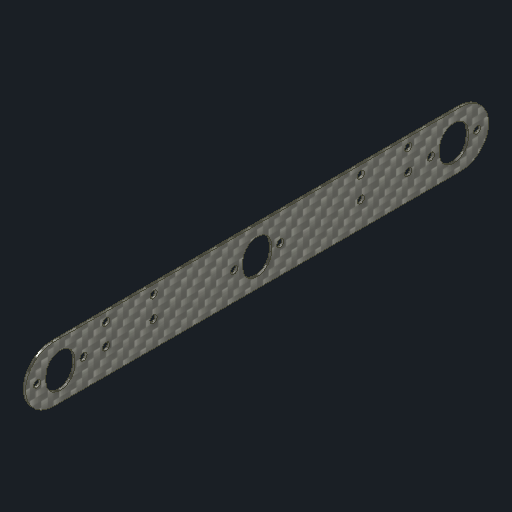
# Autodesk Inventor part: Leg_Loadpipe_Plate_Inner
Saved by Autodesk Inventor 2024.1 (Build 281209000, 209)
## iProperties
Created: 2023-06-16
Part Number: Leg_Loadpipe_Plate_Inner
Material: CFRP
Document SubType Name: Modeling
Designer: dzw04
Density: 1.43 g/cm^3
Appearance: Carbon Fiber 1
Author: dzw04
Autodesk Inventor part; units mm, degrees
ref_plane "YZ Plane" through (0, 0, 0) normal (1, 0, 0) x (0, 1, 0)
ref_plane "XZ Plane" through (0, 0, 0) normal (0, 1, 0) x (-1, 0, 0)
ref_plane "XY Plane" through (0, 0, 0) normal (0, 0, 1) x (1, 0, 0)
sketch "Sketch1" plane through (0, 0, 0) normal (1, 0, 0) x (0, 1, 0)
  line L0 (-1.25, 6.25) -> (1.25, 6.25)
  arc A0 (1.25, -6.25) -> (1.25, 6.25) centre (1.25, 0) ccw
  line L1 (1.25, -6.25) -> (-1.25, -6.25)
  arc A1 (-1.25, 6.25) -> (-1.25, -6.25) centre (-1.25, 0) ccw
  circle A2 centre (0, -10) radius 1.6
  circle A3 centre (0, 10) radius 1.6
  circle A4 centre (8.25, 44.75) radius 1.6
  circle A5 centre (8.25, 65.25) radius 1.6
  line L2 (-1.25, 91.25) -> (1.25, 91.25)
  arc A6 (1.25, 78.75) -> (1.25, 91.25) centre (1.25, 85) ccw
  line L3 (1.25, 78.75) -> (-1.25, 78.75)
  arc A7 (-1.25, 91.25) -> (-1.25, 78.75) centre (-1.25, 85) ccw
  circle A8 centre (0, 75) radius 1.6
  circle A9 centre (0, 95) radius 1.6
  line L4 (-1.25, -91.25) -> (1.25, -91.25)
  arc A10 (1.25, -91.25) -> (1.25, -78.75) centre (1.25, -85) ccw
  line L5 (1.25, -78.75) -> (-1.25, -78.75)
  arc A11 (-1.25, -78.75) -> (-1.25, -91.25) centre (-1.25, -85) ccw
  circle A12 centre (0, -75) radius 1.6
  circle A13 centre (0, -95) radius 1.6
  circle A14 centre (-0.972, 44.75) radius 1.6
  circle A15 centre (-0.972, 65.25) radius 1.6
  circle A16 centre (8.25, -44.75) radius 1.6
  circle A17 centre (8.25, -65.25) radius 1.6
  circle A18 centre (-0.972, -44.75) radius 1.6
  circle A19 centre (-0.972, -65.25) radius 1.6
  arc A20 (12, 88) -> (-12, 88) centre (0, 88) ccw
  line L6 (12, 88) -> (12, -88)
  arc A21 (-12, -88) -> (12, -88) centre (0, -88) ccw
  line L7 (-12, -88) -> (-12, 88)
  point P0 (0, 0)
  point P1 (0, 0)
  point P2 (-12, -88)
  point P3 (12, 88)
  point P4 (-12, 88)
  point P5 (1.25, -78.75)
  point P6 (1.25, 78.75)
  point P7 (-1.25, 78.75)
  point P8 (1.25, -6.25)
  point P9 (-1.25, -6.25)
  dimension "d2" = 3.2
  dimension "d3" = 3.2
  dimension "d4" = 3.2
  dimension "d5" = 3.2
  dimension "d6" = 9.222
  dimension "d7" = 9.222
  dimension "d8" = 9.222
  dimension "d11" = 3.2
  dimension "d12" = 3.2
  dimension "d13" = 3.2
  dimension "d14" = 3.2
  dimension "d15" = 3.2
  dimension "d16" = 3.2
  dimension "d17" = 3.2
  dimension "d18" = 3.2
  dimension "d19" = 3.2
  dimension "d20" = 3.2
  constraints: 22 centre point, 16 end point, 16 point on circle, 6 horizontal, 4 horizontal alignment, 2 vertical, 1 vertical alignment, 60 other
  measures "d2" diameter of A15
  measures "d3" diameter of A14
  measures "d4" diameter of A18
  measures "d5" diameter of A19
  measures "d6" distance of A19.centre A17.centre
  measures "d7" distance of A18.centre A16.centre
  measures "d8" distance of A14.centre A4.centre
  measures "d11" diameter of A5
  measures "d12" diameter of A4
  measures "d13" diameter of A16
  measures "d14" diameter of A17
  measures "d15" diameter of A9
  measures "d16" diameter of A8
  measures "d17" diameter of A3
  measures "d18" diameter of A2
  measures "d19" diameter of A12
  measures "d20" diameter of A13
extrude "Extrusion1" add sketch "Sketch1" along normal blind 1
equation "\"d7\" = d6"
equation "\"d8\" = d6"
body "Solid1"
